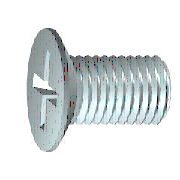
# Autodesk Inventor part: AS 1427 - M5 x 16
Saved by Autodesk Inventor 2023.2 (Build 272271000, 271)
## iProperties
Created: 2022-02-04
Part Number: AS 1427 - M5 x 16
Material: Steel, Mild
Description: Pozidriv ISO metric machine screws
Document SubType Name: Modeling
Standard: AS 1427
Designer: remop
Standards Organization: AS
Language: en-US
Size Designation: M5 x 16
Categories: <MemberInstance><Categories><Category DisplayName="Fasteners" InternalName="e4da775c-781d-43d5-af7c-5136215cf5a6" Mnemonic="FSTN"><Category DisplayName="Bolts" InternalName="536e6df0-f778-49ac-b2f2-25c71d2aa0b2" Mnemonic="SCRW"><CategoryParameter DisplayName="Nominal Diameter Designation" InternalName="03caf894-eafd-4c09-a035-916ac084b87b" Mnemonic="nomdiadesig"/><CategoryParameter DisplayName="Nominal Length" InternalName="238ecbaf-3e6c-45dd-aa95-4068c8e0fd02" Mnemonic="nomlen"/><CategoryParameter DisplayName="Thread Designation" InternalName="586d5e89-370a-4089-914f-0110033585c7" Mnemonic="thrdesign"/><CategoryParameter DisplayName="Thread Series Designation" InternalName="87c5849c-b3a5-4c3e-9c9b-2feecef9be86" Mnemonic="thrserdsgn"/><CategoryParameter DisplayName="Nominal Diameter" InternalName="8bbe3f8e-44cf-40a9-a251-3a6edc8168d6" Mnemonic="nomdia"/><CategoryParameter DisplayName="Thread Type" InternalName="b4bbb7bc-d6aa-4c9f-a9a9-4152b9f6fe49" Mnemonic="thrtype"/><CategoryParameter DisplayName="Thread Pitch" InternalName="bb82302e-82d8-4176-8fc1-c5d7bb17d5ad" Mnemonic="pitch1"/><CategoryParameter DisplayName="Threads per Unit" InternalName="bdc6e7d2-ffd0-4d9c-a173-16b95ebb912d" Mnemonic="thrperunit1"/><CategoryParameter DisplayName="Thread Class" InternalName="ebc0d23b-2cc6-4d2a-b376-d52aae53bab6" Mnemonic="thrclss"/><Category DisplayName="Countersunk" InternalName="49656530-5684-4604-a233-68d537625f23" Mnemonic="CSSCRW"><CategoryParameter DisplayName="Type" InternalName="161b33bb-bee3-4fab-a17d-97511dff40f0" Mnemonic="type"/><CategoryParameter DisplayName="Thread Length" InternalName="207f0278-6dec-43ab-bffc-1c6d03e64de4" Mnemonic="thrlen"/><CategoryParameter DisplayName="Grip Length" InternalName="2fff3de5-ce2a-45fd-9425-99ddc9dff352" Mnemonic="grplen"/><CategoryParameter DisplayName="Property Class" InternalName="5249b721-5ecc-4781-a2e8-d7e3bda3ecca" Mnemonic="propclss"/><CategoryParameter DisplayName="Head Height" InternalName="57526df9-da71-45fb-acb4-1d0529a34778" Mnemonic="headh"/><CategoryParameter DisplayName="Shank Diameter" InternalName="7ece923f-d8ee-40d5-83f8-980cad520964" Mnemonic="grpdia"/><CategoryParameter DisplayName="Head Diameter" InternalName="a509cd31-06d1-44c5-b54e-d7a695352906" Mnemonic="headdia"/><CategoryParameter DisplayName="Head Angle" InternalName="dbcfc1e0-7990-403e-bc2e-90d1c639222a" Mnemonic="headang"/></Category></Category></Category><Category DisplayName="DataType" InternalName="23b78d0f-2648-40c6-8793-ca6db495c9e8" Mnemonic="DATATYPE"><CategoryParameter DisplayName="DisplayName" InternalName="05415f3d-3907-474b-a020-eb9d644f4cf3" Mnemonic="DISPLAYNAME"/><CategoryParameter DisplayName="Standard" InternalName="0c0a119c-1e12-4c84-803f-101930972f5e" Mnemonic="STANDARD"/><CategoryParameter DisplayName="Description" InternalName="13903e3d-64b1-4950-80da-f627842ea37f" Mnemonic="DESCRIPTION"/><CategoryParameter DisplayName="Designation" InternalName="2675968c-4ce5-49e0-a4f5-552d29089031" Mnemonic="DESIGNATION"/><CategoryParameter DisplayName="Default Row" InternalName="2af9ec52-faaa-4026-b378-f9fa4afca842" Mnemonic="DEFAULTROW"/><CategoryParameter DisplayName="Folder Name" InternalName="3f06958e-8713-4116-9be7-ed6184ecc97b" Mnemonic="FOLDERNAME"/><CategoryParameter DisplayName="Revision Guid" InternalName="45a75005-10b1-4dfc-8d6d-dfe629f0b93c" Mnemonic="REVISIONGUID"/><CategoryParameter DisplayName="FileName" InternalName="8b46a4cc-9585-4fed-90c3-899f57e09a73" Mnemonic="FILENAME"/><CategoryParameter DisplayName="StdsOrg" InternalName="8f5914e1-4693-403f-8ab5-d37768198c9d" Mnemonic="STDSORG"/><CategoryParameter DisplayName="Family Version" InternalName="914462f6-6e19-4b14-ba84-155b9680b1d0" Mnemonic="FAMILYREVISION"/><CategoryParameter DisplayName="Standard Revision" InternalName="91d5a463-65c2-4fde-b823-3b7fea5e8e17" Mnemonic="STANDARDREVISION"/><CategoryParameter DisplayName="Member Revision" InternalName="a65d44b9-392f-4f4f-857b-e4b3d54996fe" Mnemonic="MEMBERREVISION"/><CategoryParameter DisplayName="ClipFormat" InternalName="bc51e27b-3422-4e78-93ef-cec197ddf230" Mnemonic="CLIPFORMAT"/><CategoryParameter DisplayName="Manufacturer" InternalName="cd6c7a72-a28a-4e50-99a9-2c7f4e13e5ad" Mnemonic="MANUFACTURER"/><CategoryParameter DisplayName="InternalName" InternalName="cf1d0246-76d9-4b4a-8305-fa0409afb5c1" Mnemonic="INTERNALNAME"/><CategoryParameter DisplayName="IsMetric" InternalName="e2385c5b-1ea4-4823-96a8-8de651266ec3" Mnemonic="ISMETRIC"/><Category DisplayName="Part" InternalName="c0e0b642-3bcb-4cc8-9e80-f96d35c4afa4" Mnemonic="PART"><CategoryParameter DisplayName="Part Number" InternalName="016b6077-bfbe-49bd-92c9-d8d59c39c941" Mnemonic="PARTNUMBER"/><CategoryParameter DisplayName="Stock Number" InternalName="4dba7c1c-e26c-444e-836c-b08b433409a8" Mnemonic="STOCKNUMBER"/><CategoryParameter DisplayName="Material Key" InternalName="5c9a8adb-dd2b-4535-b97f-0a94a95fe41f" Mnemonic="MATERIALKEY"/><CategoryParameter DisplayName="Material" InternalName="818a152a-d3c3-49ca-80ee-df7d91421b8e" Mnemonic="MATERIAL"/></Category></Category><Category DisplayName="LegacyMap" InternalName="cd87c42b-3e48-431e-b5c0-1cbeb14dfe77" Mnemonic="LEGACYMAP"><CategoryParameter DisplayName="unique DA member ID" InternalName="0918ad47-427f-4fed-ae26-24c81c58f590" Mnemonic="DACOOKIE"/><CategoryParameter DisplayName="Merge11 ID" InternalName="0ee8fb18-e2ed-4f39-96f6-1f4b5f50aa71" Mnemonic="MERGE11"/><CategoryParameter DisplayName="unique CC member ID" InternalName="5193edd4-b2b0-4ab4-9d54-de900eee34e0" Mnemonic="CCCOOKIE"/><CategoryParameter DisplayName="Split ID" InternalName="72b5c83c-be7f-45c4-ae51-9160ea6deb26" Mnemonic="SPLIT"/><CategoryParameter DisplayName="MemberID" InternalName="8e5e0294-fc51-4c8f-b3d7-003dc5ed94f6" Mnemonic="MEMBERID"/><CategoryParameter DisplayName="CatalogName" InternalName="d99d1e27-aa94-4de2-af4c-c348882a6f4f" Mnemonic="CATALOGNAME"/><CategoryParameter DisplayName="FamilyNumber" InternalName="e705e1f4-09cb-413e-91f9-551b4188271e" Mnemonic="FAMILYNUMBER"/></Category></Categories><FamilyTemplate Id="si0140"><FamilyTemplateParameters><FamilyTemplateParameter ObjectType="kUserParameterObject" ValueType="xs:double" Id="1" ObjectReferenceKey="GUL"/><FamilyTemplateParameter ObjectType="kUserParameterObject" ValueType="xs:double" Id="2" ObjectReferenceKey="SPD"/><FamilyTemplateParameter ObjectType="kUserParameterObject" ValueType="xs:double" Id="3" ObjectReferenceKey="NLG"/><FamilyTemplateParameter ObjectType="kUserParameterObject" ValueType="xs:double" Id="4" ObjectReferenceKey="KOD"/><FamilyTemplateParameter ObjectType="kUserParameterObject" ValueType="xs:double" Id="5" ObjectReferenceKey="SBR"/><FamilyTemplateParameter ObjectType="kUserParameterObject" ValueType="xs:double" Id="6" ObjectReferenceKey="TOA"/><FamilyTemplateParameter ObjectType="kUserParameterObject" ValueType="xs:double" Id="7" ObjectReferenceKey="SDM"/><FamilyTemplateParameter ObjectType="kUserParameterObject" ValueType="xs:double" Id="8" ObjectReferenceKey="EPV"/><FamilyTemplateParameter ObjectType="kUserParameterObject" ValueType="xs:double" Id="9" ObjectReferenceKey="THREADDIA"/><FamilyTemplateParameter ObjectType="kUserParameterObject" ValueType="xs:double" Id="10" ObjectReferenceKey="GEL"/><FamilyTemplateParameter ObjectType="kUserParameterObject" ValueType="xs:double" Id="11" ObjectReferenceKey="INTI"/><FamilyTemplateParameter ObjectType="kUserParameterObject" ValueType="xs:double" Id="12" ObjectReferenceKey="BDM"/><FamilyTemplateParameter ObjectType="kUserParameterObject" ValueType="xs:double" Id="13" ObjectReferenceKey="RR"/><FamilyTemplateParameter ObjectType="kUserParameterObject" ValueType="xs:double" Id="14" ObjectReferenceKey="KOH"/><FamilyTemplateParameter ObjectType="kUserParameterObject" ValueType="xs:double" Id="15" ObjectReferenceKey="TPU"/><FamilyTemplateParameter ObjectType="kUserParameterObject" ValueType="xs:double" Id="16" ObjectReferenceKey="PTC"/><FamilyTemplateParameter ObjectType="kUserParameterObject" ValueType="xs:double" Id="17" ObjectReferenceKey="NND"/><FamilyTemplateParameter ObjectType="kUserParameterObject" ValueType="xs:double" Id="18" ObjectReferenceKey="GD"/><FamilyTemplateParameter ObjectType="kUserParameterObject" ValueType="xs:double" Id="19" ObjectReferenceKey="SEWI"/><FamilyTemplateParameter ObjectType="kUserParameterObject" ValueType="xs:double" Id="20" ObjectReferenceKey="GAL"/><FamilyTemplateParameter ObjectType="kUserParameterObject" ValueType="xs:double" Id="21" ObjectReferenceKey="GD1"/><FamilyTemplateParameter ObjectType="kPropertyObject" ValueType="xs:string" Id="100" ObjectReferenceKey="{32853F0F-3444-11d1-9E93-0060B03C1CA6}" SubObjectId="52"/><FamilyTemplateParameter ObjectType="kPropertyObject" ValueType="xs:string" Id="105" ObjectReferenceKey="{32853F0F-3444-11d1-9E93-0060B03C1CA6}" SubObjectId="5"/><FamilyTemplateParameter ObjectType="kPartComponentDefinitionObject" ValueType="xs:string" Id="110" SubObjectId="Material"/><FamilyTemplateParameter ObjectType="kThreadFeatureObject" ValueType="xs:structure" Id="300" ObjectReferenceKey="1002000010000000ed150000000000008000000000000000" SubObjectId="ThreadInfo"><FamilyTemplateParameter ObjectType="" ValueType="xs:string" Id="301" SubObjectId="ThreadDesignation"/><FamilyTemplateParameter ObjectType="" ValueType="xs:string" Id="302" SubObjectId="ThreadType"/><FamilyTemplateParameter ObjectType="" ValueType="xs:string" Id="303" SubObjectId="ThreadClass"/></FamilyTemplateParameter></FamilyTemplateParameters></FamilyTemplate><CategoryParameterMap><ParamToTemplateMap><ParamToTemplate CategoryParameter="//CategoryParameter[@InternalName='05415f3d-3907-474b-a020-eb9d644f4cf3']" ConstantValue="AS 1427 H - Metric"/><ParamToTemplate CategoryParameter="//CategoryParameter[@InternalName='cf1d0246-76d9-4b4a-8305-fa0409afb5c1']" ConstantValue="6709d4e1-e633-491e-a295-a3190630f03f"/><ParamToTemplate CategoryParameter="//CategoryParameter[@InternalName='3f06958e-8713-4116-9be7-ed6184ecc97b']" ConstantValue="AS 1427(04)"/><ParamToTemplate CategoryParameter="//CategoryParameter[@InternalName='914462f6-6e19-4b14-ba84-155b9680b1d0']" ConstantValue="10"/><ParamToTemplate CategoryParameter="//CategoryParameter[@InternalName='bc51e27b-3422-4e78-93ef-cec197ddf230']" ConstantValue="CF_INVENTOR.STDPARTS"/><ParamToTemplate CategoryParameter="//CategoryParameter[@InternalName='e2385c5b-1ea4-4823-96a8-8de651266ec3']" ConstantValue="true"/><ParamToTemplate CategoryParameter="//CategoryParameter[@InternalName='13903e3d-64b1-4950-80da-f627842ea37f']" ConstantValue="Pozidriv ISO metric machine screws"/><ParamToTemplate CategoryParameter="//CategoryParameter[@InternalName='8f5914e1-4693-403f-8ab5-d37768198c9d']" ConstantValue="AS"/><ParamToTemplate CategoryParameter="//CategoryParameter[@InternalName='0c0a119c-1e12-4c84-803f-101930972f5e']" ConstantValue="AS 1427"/><ParamToTemplate CategoryParameter="//CategoryParameter[@InternalName='cd6c7a72-a28a-4e50-99a9-2c7f4e13e5ad']" TemplateParameter="104"/><ParamToTemplate CategoryParameter="//CategoryParameter[@InternalName='91d5a463-65c2-4fde-b823-3b7fea5e8e17']" TemplateParameter="103"/><ParamToTemplate CategoryParameter="//CategoryParameter[@InternalName='45a75005-10b1-4dfc-8d6d-dfe629f0b93c']" ConstantValue="9a45f60e-164f-4d3f-bbb8-41462dfe9aff"/><ParamToTemplate CategoryParameter="//CategoryParameter[@InternalName='2af9ec52-faaa-4026-b378-f9fa4afca842']" ConstantValue="10"/><ParamToTemplate CategoryParameter="//CategoryParameter[@InternalName='d99d1e27-aa94-4de2-af4c-c348882a6f4f']" ConstantValue="AS"/><ParamToTemplate CategoryParameter="//CategoryParameter[@InternalName='e705e1f4-09cb-413e-91f9-551b4188271e']" ConstantValue="2"/><ParamToTemplate CategoryParameter="//CategoryParameter[@InternalName='8b46a4cc-9585-4fed-90c3-899f57e09a73']" ConstantValue="AS 1427 - M5 x 16(5) I"/><ParamToTemplate CategoryParameter="//CategoryParameter[@InternalName='a65d44b9-392f-4f4f-857b-e4b3d54996fe']" ConstantValue="3A25DAA9-9540-4BE2-8FC0-4BA92714BF4C"/><ParamToTemplate CategoryParameter="//CategoryParameter[@InternalName='2fff3de5-ce2a-45fd-9425-99ddc9dff352']" ConstantValue="4.1"/><ParamToTemplate CategoryParameter="//CategoryParameter[@InternalName='ebc0d23b-2cc6-4d2a-b376-d52aae53bab6']" ConstantValue="6g"/><ParamToTemplate CategoryParameter="//CategoryParameter[@InternalName='03caf894-eafd-4c09-a035-916ac084b87b']" ConstantValue="M5"/><ParamToTemplate CategoryParameter="//CategoryParameter[@InternalName='b4bbb7bc-d6aa-4c9f-a9a9-4152b9f6fe49']" ConstantValue="ISO Metric profile"/><ParamToTemplate CategoryParameter="//CategoryParameter[@InternalName='8e5e0294-fc51-4c8f-b3d7-003dc5ed94f6']" ConstantValue="630"/><ParamToTemplate CategoryParameter="//CategoryParameter[@InternalName='7ece923f-d8ee-40d5-83f8-980cad520964']" TemplateParameter="12"/><ParamToTemplate CategoryParameter="//CategoryParameter[@InternalName='2675968c-4ce5-49e0-a4f5-552d29089031']" TemplateParameter="100"/><ParamToTemplate CategoryParameter="//CategoryParameter[@InternalName='207f0278-6dec-43ab-bffc-1c6d03e64de4']" TemplateParameter="10"/><ParamToTemplate CategoryParameter="//CategoryParameter[@InternalName='a509cd31-06d1-44c5-b54e-d7a695352906']" TemplateParameter="4"/><ParamToTemplate CategoryParameter="//CategoryParameter[@InternalName='57526df9-da71-45fb-acb4-1d0529a34778']" TemplateParameter="14"/><ParamToTemplate CategoryParameter="//CategoryParameter[@InternalName='818a152a-d3c3-49ca-80ee-df7d91421b8e']" TemplateParameter="110"/><ParamToTemplate CategoryParameter="//CategoryParameter[@InternalName='238ecbaf-3e6c-45dd-aa95-4068c8e0fd02']" TemplateParameter="3"/><ParamToTemplate CategoryParameter="//CategoryParameter[@InternalName='8bbe3f8e-44cf-40a9-a251-3a6edc8168d6']" TemplateParameter="17"/><ParamToTemplate CategoryParameter="//CategoryParameter[@InternalName='016b6077-bfbe-49bd-92c9-d8d59c39c941']" TemplateParameter="105"/><ParamToTemplate CategoryParameter="//CategoryParameter[@InternalName='bb82302e-82d8-4176-8fc1-c5d7bb17d5ad']" TemplateParameter="16"/><ParamToTemplate CategoryParameter="//CategoryParameter[@InternalName='dbcfc1e0-7990-403e-bc2e-90d1c639222a']" TemplateParameter="19"/><ParamToTemplate CategoryParameter="//CategoryParameter[@InternalName='586d5e89-370a-4089-914f-0110033585c7']" TemplateParameter="301"/><ParamToTemplate CategoryParameter="//CategoryParameter[@InternalName='bdc6e7d2-ffd0-4d9c-a173-16b95ebb912d']" TemplateParameter="15"/></ParamToTemplateMap></CategoryParameterMap></MemberInstance>
Density: 7.85 g/cm^3
Appearance: Semi-Polished
IsCustomPart: 0
Author: remop
Autodesk Inventor part; units mm, degrees
ref_plane "YZ Plane" through (0, 0, 0) normal (1, 0, 0) x (0, 1, 0)
ref_plane "XZ Plane" through (0, 0, 0) normal (0, 1, 0) x (-1, 0, 0)
sketch "Sketch1" plane through (0, 0, 0) normal (0, 0, 1) x (1, 0, 0)
  line L0 (2.05, 0) -> (16, 0)
  line L1 (16, 0) -> (16, 2.5)
  line L2 (16, 2.5) -> (4.1, 2.5)
  line L3 (4.1, 2.5) -> (3.6092, 2.2546)
  line L4 (3.6092, 2.2546) -> (2.5, 2.2546)
  line L5 (0, 4.4) -> (0, 2.21)
  line L6 (0, 2.21) -> (1.1905, 1.6164)
  line L7 (1.1905, 1.6164) -> (2.05, 0)
  line L8 (-3.2, 0) -> (19.2, 0) projected
  line L9 (0, -0.88) -> (0, 5.28) projected
  line L10 (0, 4.4) -> (0.3546, 4.4)
  line L11 (0.3546, 4.4) -> (2.5, 2.2546)
  line L12 (4.1, 2.5) -> (2.2546, 2.5) construction
  dimension "d1" = 11.9
  dimension "d2" = 5
  dimension "d3" = 4.5092
  dimension "d4" = 4.42
  dimension "d5" = 26.5
  dimension "d6" = 62
  dimension "d7" = 2.05
  dimension "d8" = 0.4908
  dimension "d12" = 8.8
  dimension "d13" = 45
  dimension "d15" = 16
  dimension "d24" = 2.5
  constraints: 22 end point, 3 parallel, 3 perpendicular, 2 collinear, 1 horizontal, 1 point on line
  measures "d1" distance of L1.end L2.end
  measures "d2" diameter of L2 L0
  measures "d3" diameter of L4 L0
  measures "d4" diameter of L5.end L0
  measures "d5" angle of L6 L0
  measures "d6" angle of L7 L0
  measures "d7" distance from line of L0.start L5
  measures "d8" horizontal distance of L3.end L2.end
  measures "d12" diameter of L10 L0
  measures "d13" angle of L11 L0
  measures "d15" distance between parallel lines of L1 L5
  measures "d24" distance from line of L4.end L5
revolve "Body" add sketch "Sketch1" angle 360 about axis through (2.05, 0, 0) along (1, 0, 0) contours L7 L6 L5 L10 L11 L4 L3 L2 L1 L0
sketch "Sketch2" plane through (0, 0, 0) normal (-1, 0, 0) x (0, 0, 1)
  line L0 (0, 2.21) -> (0, 0) construction
  line L1 (0, 0) -> (2.21, 0) construction
  arc A0 (0.663, 0) -> (0, 0.663) centre (0, 0) ccw construction
  arc A1 (0.7735, 0) -> (0, 0.7735) centre (0, 0) ccw construction
  arc A2 (2.1539, 0.495) -> (0.495, 2.1539) centre (0, 0) ccw
  line L2 (0, 0) -> (1.5627, 1.5627) construction
  line L3 (0.495, 2.1539) -> (0.3952, 0.6649)
  line L4 (2.1539, 0.495) -> (0.6649, 0.3952)
  arc A3 (0.495, 2.1539) -> (0, 2.21) centre (0, 0) ccw
  arc A4 (2.21, 0) -> (2.1539, 0.495) centre (0, 0) ccw
  line L5 (0, -6.16) -> (0, 6.16) projected
  line L6 (-6.16, 0) -> (6.16, 0) projected
  arc A5 (0.495, -2.1539) -> (2.1539, -0.495) centre (0, 0) ccw
  line L7 (0.495, -2.1539) -> (0.3952, -0.6649)
  line L8 (2.1539, -0.495) -> (0.6649, -0.3952)
  arc A6 (0, -2.21) -> (0.495, -2.1539) centre (0, 0) ccw
  arc A7 (2.1539, -0.495) -> (2.21, 0) centre (0, 0) ccw
  arc A8 (-0.495, 2.1539) -> (-2.1539, 0.495) centre (0, 0) ccw
  line L9 (-0.495, 2.1539) -> (-0.3952, 0.6649)
  line L10 (-2.1539, 0.495) -> (-0.6649, 0.3952)
  arc A9 (0, 2.21) -> (-0.495, 2.1539) centre (0, 0) ccw
  arc A10 (-2.1539, 0.495) -> (-2.21, 0) centre (0, 0) ccw
  arc A11 (-0.495, -2.1539) -> (0, -2.21) centre (0, 0) ccw
  arc A12 (-2.1539, -0.495) -> (-0.495, -2.1539) centre (0, 0) ccw
  arc A13 (-2.21, 0) -> (-2.1539, -0.495) centre (0, 0) ccw
  line L11 (-2.1539, -0.495) -> (-0.6649, -0.3952)
  line L12 (-0.495, -2.1539) -> (-0.3952, -0.6649)
  arc A14 (0.3952, 0.6649) -> (0.6649, 0.3952) centre (0.648, 0.648) ccw
  arc A15 (0.6649, -0.3952) -> (0.3952, -0.6649) centre (0.648, -0.648) ccw
  arc A16 (-0.6649, 0.3952) -> (-0.3952, 0.6649) centre (-0.648, 0.648) ccw
  arc A17 (-0.3952, -0.6649) -> (-0.6649, -0.3952) centre (-0.648, -0.648) ccw
  point P0 (1.5627, -1.5627)
  point P1 (-1.5627, 1.5627)
  point P2 (-1.5627, -1.5627)
  dimension "d17" = 1.326
  dimension "d18" = 1.547
  dimension "d19" = 4.42
  dimension "d20" = 45
  dimension "d21" = 0.495
  constraints: 41 point on circle, 22 end point, 22 symmetric about line, 18 centre point, 11 coincident, 4 point on line, 3 tangent, 2 collinear, 1 perpendicular, 1 vertical, 19 other
  measures "d17" diameter of A0
  measures "d18" diameter of A1
  measures "d19" diameter of A2
  measures "d20" angle of L2 L1
  measures "d21" distance from line of L3.start L0
extrude "Slot" add sketch "Sketch2" against normal up to next draft 5 contours L4 A14 L3 A2 | A5 L7 A15 L8 | L9 A16 L10 A8 | A12 L11 A17 L12
fillet "Fillet1" radius 0.198 4 edges at (0, 2.21, 0) (0, 0, -2.21) (0, -2.21, 0) (0, 0, 2.21)
thread "Thread" size "M5x0.8" class "6g" standard "ISO Metric profile" length 11.9
chamfer "Chamfer1" distance 0.4908 distance2 0.2454 1 edges at (16, -2.5, 0) measured on face at (16, 0.2278, 0.5045)
ref_plane "Work Plane2" through (3.35, 0, 0) normal (0, 0, -1) x (1, 0, 0)
equation "\"d1\" = GEL"
equation "\"d2\" = GD"
equation "\"d3\" = BDM"
equation "\"d4\" = SDM"
equation "\"d7\" = INTI"
equation "\"d8\" = GAL"
equation "\"d12\" = KOD"
equation "\"d13\" = 0.5 * SEWI"
equation "\"d15\" = NLG"
equation "\"d24\" = KOH"
equation "\"d17\" = 0.3 * SDM"
equation "\"d18\" = 0.35 * SDM"
equation "\"d19\" = SDM"
equation "\"d21\" = 0.5 * SBR"
equation "\"d23\" = 0.2 * SBR"
equation "\"d10\" = GEL"
equation "\"d25\" = -0.5 * SPD + 0.5 * GD"
equation "\"d26\" = 0.5 * GAL"
equation "\"NLG\" = 16"
equation "\"GEL\" = 11.9"
equation "\"GAL\" = 0.61345 * PTC"
equation "\"SPD\" = NND - 1.2269 * PTC"
equation "\"KOD\" = 8.8"
equation "\"KOH\" = 2.5"
equation "\"SBR\" = 0.99"
equation "\"INTI\" = 2.05"
equation "\"SDM\" = 4.42"
equation "\"GD\" = NND"
equation "\"BDM\" = NND - GAL"
equation "\"SEWI\" = 90deg"
equation "\"d9\" = SDM"
equation "\"GUL\" = 0.61345 * PTC"
equation "\"TOA\" = 30deg"
equation "\"EPV\" = 5"
equation "\"THREADDIA\" = 5"
equation "\"RR\" = 0.5"
equation "\"PTC\" = 0.8"
equation "\"NND\" = 5"
equation "\"GD1\" = THREADDIA - 1.2269 * PTC"
body "Solid1"
